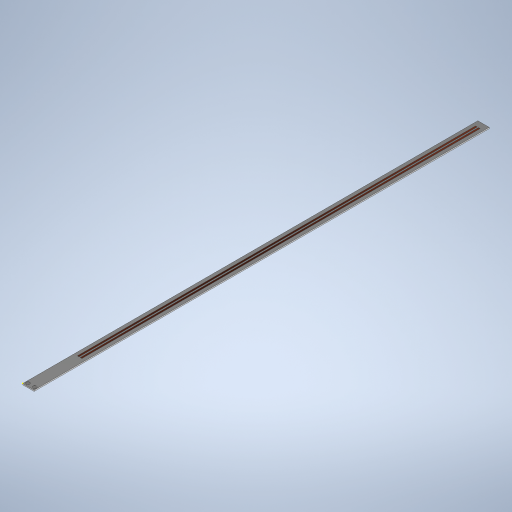
# Autodesk Inventor part: Dosyn Rail
Saved by Autodesk Inventor 2024 (Build 280153000, 153)
## iProperties
Created: 2023-11-15
Part Number: Dosyn Rail
Material: 常规
Document SubType Name: Sheet Metal
Designer: lunima
Density: 1 g/cm^3
Sheet Metal Rule: 默认_mm
Appearance: 默认
Author: lunima
Autodesk Inventor part; units mm, degrees
ref_plane "YZ Plane" through (0, 0, 0) normal (1, 0, 0) x (0, 1, 0)
ref_plane "XZ Plane" through (0, 0, 0) normal (0, 1, 0) x (-1, 0, 0)
ref_plane "XY Plane" through (0, 0, 0) normal (0, 0, 1) x (1, 0, 0)
sketch "草图1" plane through (0, 0, 0) normal (0, 1, 0) x (-1, 0, 0)
  line L0 (0, 0) -> (-10, 0)
  line L1 (-10, 0) -> (-10, -400)
  line L2 (-10, -400) -> (0, -400)
  line L3 (0, -400) -> (0, 0)
  dimension "d0" = 10
  dimension "d1" = 400
  constraints: 8 end point, 2 parallel, 1 horizontal, 1 perpendicular
  measures "d0" distance of L2.end L1.end
  measures "d1" distance of L1.end L0.end
extrude "拉伸1" add sketch "草图1" along normal blind 1
sketch "草图2" plane through (0, 1, 0) normal (0, 1, 0) x (1, 0, 0)
  circle A0 centre (2, 2.5) radius 1.5
  circle A1 centre (8, 2.5) radius 1.5
  line L0 (0, 400) -> (0, 0) projected
  line L1 (10, 0) -> (10, 400) projected
  line L2 (0, 0) -> (10, 0) projected
  dimension "d4" = 3
  dimension "d5" = 3
  dimension "d6" = 2
  dimension "d7" = 2
  dimension "d8" = 2.5
  dimension "d9" = 2.5
  constraints: 2 centre point
  measures "d4" diameter of A0
  measures "d5" diameter of A1
  measures "d6" distance from line of L0 A0.centre
  measures "d7" distance from line of L1 A1.centre
  measures "d8" distance from line of L2 A1.centre
  measures "d9" distance from line of L2 A0.centre
sketch "草图3" plane through (0, 1, 0) normal (0, 1, 0) x (1, 0, 0)
  point P0 (0, 0)
extrude "拉伸2" add sketch "草图2" along normal blind 0.1
sketch "草图4" plane through (2, 1.1, -2.5) normal (0, 1, 0) x (1, 0, 0)
  circle A0 centre (0, 0) radius 1.5 projected
  circle A1 centre (0, 0) radius 0.75
  circle A2 centre (6, 0) radius 1.5 projected
  circle A3 centre (6, 0) radius 0.75
  point P0 (-2, -2.5)
  dimension "d12" = 1.5
  dimension "d13" = 1.5
  constraints: 2 centre point, 2 coincident
  measures "d12" diameter of A1
  measures "d13" diameter of A3
extrude "拉伸3" cut sketch "草图4" against normal blind 3.85 contours A1 | A3
sketch "草图5" plane through (0, 1, 0) normal (0, 1, 0) x (1, 0, 0)
  line L0 (3.0005, 45) -> (4.4505, 45)
  line L1 (4.4505, 45) -> (4.4505, 395)
  line L2 (4.4505, 395) -> (3.0005, 395)
  line L3 (3.0005, 395) -> (3.0005, 45)
  line L4 (5.5405, 45) -> (6.9905, 45)
  line L5 (6.9905, 45) -> (6.9905, 395)
  line L6 (6.9905, 395) -> (5.5405, 395)
  line L7 (5.5405, 395) -> (5.5405, 45)
  line L8 (0, 0) -> (10, 0) projected
  line L9 (10, 400) -> (0, 400) projected
  line L10 (0, 400) -> (0, 0) projected
  dimension "d16" = 1.45
  dimension "d17" = 350
  dimension "d18" = 1.45
  dimension "d19" = 350
  dimension "d20" = 45
  dimension "d21" = 5
  dimension "d22" = 1.09
  dimension "d23" = 3.0005
  constraints: 16 end point, 4 parallel, 2 horizontal, 2 perpendicular, 1 point on line
  measures "d16" distance of L2.end L1.end
  measures "d17" distance of L1.end L0.end
  measures "d18" distance of L6.end L5.end
  measures "d19" distance of L5.end L4.end
  measures "d20" distance between parallel lines of L8 L0
  measures "d21" distance between parallel lines of L2 L9
  measures "d22" distance between parallel lines of L7 L1
  measures "d23" distance between parallel lines of L10 L3
extrude "拉伸4" add sketch "草图5" along normal blind 0.1
equation "\"折弯半径\" = 厚度"
equation "\"折弯释压宽度\" = 厚度"
equation "\"折弯释压深度\" = 0.5 * 厚度"
equation "\"拐角释压尺寸\" = 4 * 厚度"
equation "\"最小余量\" = 2 * 厚度"
equation "\"过渡半径\" = 折弯半径"
equation "\"Jacobi半径尺寸\" = 折弯半径"
equation "\"间隙大小\" = 厚度"
equation "\"厚度\" = 0.5"
